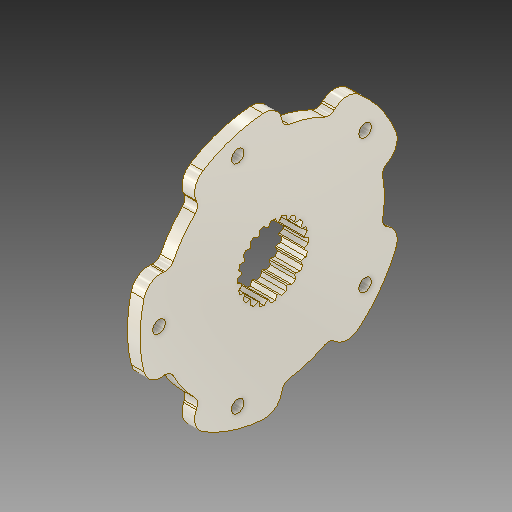
# Autodesk Inventor part: 362-04
Saved by Autodesk Inventor 2019 (Build 230136000, 136)
## iProperties
Company: Autodesk Inc.
Created: 2017-03-19
Part Number: 362-04
Material: Titanium
Document SubType Name: Modeling
Designer: Autodesk Inc.
Density: 4.51 g/cm^3
Appearance: Titanium - Polished
Mass: 217.983 g
Surface Area: 181.774 cm^2
Volume: 48.3334 cm^3
Author: Inventor
Autodesk Inventor part; units mm, degrees
ref_plane "YZ Plane" through (0, 0, 0) normal (1, 0, 0) x (0, 1, 0)
ref_plane "XZ Plane" through (0, 0, 0) normal (0, 1, 0) x (-1, 0, 0)
ref_plane "XY Plane" through (0, 0, 0) normal (0, 0, 1) x (1, 0, 0)
sketch "Sketch1" plane through (0, 0, 0) normal (1, 0, 0) x (0, 1, 0)
  arc A0 (12.5, 50.9902) -> (-12.5, 50.9902) centre (0, 0) ccw
  arc A1 (-19.5, 39.443) -> (-17.7114, 42.7254) centre (-20.9403, 42.3564) ccw
  line L0 (-17.7114, 42.7254) -> (-17.7881, 43.3968)
  arc A2 (-12.5, 50.9902) -> (-17.7881, 43.3968) centre (-10.8333, 44.1915) ccw
  line L1 (0, 0) -> (0, 52.5) construction
  arc A3 (17.7881, 43.3968) -> (12.5, 50.9902) centre (10.8333, 44.1915) ccw
  line L2 (17.7114, 42.7254) -> (17.7881, 43.3968)
  arc A4 (17.7114, 42.7254) -> (19.5, 39.443) centre (20.9403, 42.3564) ccw
  arc A5 (-44.6318, 27.645) -> (-52.3573, 3.8686) centre (0, 0) ccw
  arc A6 (-43.5384, -6.357) -> (-46.1074, -3.6416) centre (-46.7543, -6.8266) ccw
  line L3 (-46.1074, -3.6416) -> (-46.7696, -3.5071)
  arc A7 (-52.3573, 3.8686) -> (-46.7696, -3.5071) centre (-45.3763, 3.3528) ccw
  line L4 (0, 0) -> (-49.9305, 16.2234) construction
  arc A8 (-35.776, 30.3278) -> (-44.6318, 27.645) centre (-38.6809, 23.959) ccw
  line L5 (-35.1611, 30.0474) -> (-35.776, 30.3278)
  arc A9 (-35.1611, 30.0474) -> (-31.4867, 30.7342) centre (-33.8124, 33.0043) ccw
  arc A10 (-40.084, -33.9046) -> (-19.8586, -48.5993) centre (0, 0) ccw
  arc A11 (-7.4082, -43.3719) -> (-10.7846, -44.976) centre (-7.9554, -46.5755) ccw
  line L6 (-10.7846, -44.976) -> (-11.1171, -45.5643)
  arc A12 (-19.8586, -48.5993) -> (-11.1171, -45.5643) centre (-17.2108, -42.1194) ccw
  line L7 (0, 0) -> (-30.8587, -42.4734) construction
  arc A13 (-39.8989, -24.6532) -> (-40.084, -33.9046) centre (-34.7395, -29.384) ccw
  line L8 (-39.4421, -24.1551) -> (-39.8989, -24.6532)
  arc A14 (-39.4421, -24.1551) -> (-38.9598, -20.4482) centre (-41.8376, -21.9586) ccw
  arc A15 (19.8586, -48.5993) -> (40.084, -33.9046) centre (0, 0) ccw
  arc A16 (38.9598, -20.4482) -> (39.4421, -24.1551) centre (41.8376, -21.9586) ccw
  line L9 (39.4421, -24.1551) -> (39.8989, -24.6532)
  arc A17 (40.084, -33.9046) -> (39.8989, -24.6532) centre (34.7395, -29.384) ccw
  line L10 (0, 0) -> (30.8587, -42.4734) construction
  arc A18 (11.1171, -45.5643) -> (19.8586, -48.5993) centre (17.2108, -42.1194) ccw
  line L11 (10.7846, -44.976) -> (11.1171, -45.5643)
  arc A19 (10.7846, -44.976) -> (7.4082, -43.3719) centre (7.9554, -46.5755) ccw
  arc A20 (52.3573, 3.8686) -> (44.6318, 27.645) centre (0, 0) ccw
  arc A21 (31.4867, 30.7342) -> (35.1611, 30.0474) centre (33.8124, 33.0043) ccw
  line L12 (35.1611, 30.0474) -> (35.776, 30.3278)
  arc A22 (44.6318, 27.645) -> (35.776, 30.3278) centre (38.6809, 23.959) ccw
  line L13 (0, 0) -> (49.9305, 16.2234) construction
  arc A23 (46.7696, -3.5071) -> (52.3573, 3.8686) centre (45.3763, 3.3528) ccw
  line L14 (46.1074, -3.6416) -> (46.7696, -3.5071)
  arc A24 (46.1074, -3.6416) -> (43.5384, -6.357) centre (46.7543, -6.8266) ccw
  arc A25 (38.9598, -20.4482) -> (43.5384, -6.357) centre (0, 0) ccw
  arc A26 (-7.4082, -43.3719) -> (7.4082, -43.3719) centre (0, 0) ccw
  arc A27 (-43.5384, -6.357) -> (-38.9598, -20.4482) centre (0, 0) ccw
  arc A28 (31.4867, 30.7342) -> (19.5, 39.443) centre (0, 0) ccw
  arc A29 (-19.5, 39.443) -> (-31.4867, 30.7342) centre (0, 0) ccw
  dimension "d118" = 52.5
  dimension "d119" = 7
  dimension "d120" = 3.25
  dimension "d121" = 360
  dimension "d122" = 44
  dimension "d123" = 12.5
  dimension "d124" = 19.5
  constraints: 77 point on circle, 30 centre point, 30 end point, 6 symmetric about line, 5 coincident, 5 tangent, 1 vertical, 142 other
  measures "d118" radius of A0
  measures "d119" radius of A2
  measures "d120" radius of A1
  measures "d122" radius of A28
  measures "d123" distance from line of L1 A0.end
  measures "d124" distance from line of L1 A1.start
extrude "Extrusion1" add sketch "Sketch1" along normal blind 5
sketch "Sketch2" plane through (0, 0, 0) normal (-1, 0, 0) x (0, 0, 1)
  circle A0 centre (0, 0) radius 32.5
  dimension "d104" = 65
  constraints: 1 centre point, 1 coincident
  measures "d104" diameter of A0
extrude "Extrusion2" add sketch "Sketch2" along normal blind 5
sketch "Sketch3" plane through (5, 0, 0) normal (1, 0, 0) x (0, 0, -1)
  line L0 (0, -73.3268) -> (0, 73.3268) construction
  line L1 (69.4432, 0) -> (-72.8239, 0) construction
  circle A0 centre (-45, 0) radius 2.5
  point P0 (0, 0)
  dimension "d107" = 5
  dimension "d108" = 45
  constraints: 1 centre point, 1 point on line
  measures "d107" diameter of A0
  measures "d108" distance from line of L0 A0.centre
extrude "Extrusion3" cut sketch "Sketch3" against normal through all
pattern_circular "Circular Pattern1" count 5 over 360 about axis through (-10, 0, 0) along (1, 0, 0) of "Extrusion3"
sketch "Sketch4" plane through (5, 0, 0) normal (1, 0, 0) x (0, 0, -1)
  arc A0 (-5.4322, 11.258) -> (-5.9149, 11.012) centre (0, 0) ccw
  line L0 (0, -21) -> (0, 21) construction
  line L1 (-0.9, 14) -> (0.9, 14)
  line L2 (-0.9, 14) -> (-1.6874, 12.3856)
  line L3 (0.9, 14) -> (1.6874, 12.3856)
  line L4 (-5.1822, 13.0367) -> (-5.4322, 11.258)
  line L5 (-5.1822, 13.0367) -> (-3.4703, 13.5929)
  line L6 (-3.4703, 13.5929) -> (-2.2225, 12.3008)
  line L7 (-8.9571, 10.7972) -> (-8.6452, 9.0283)
  line L8 (-8.9571, 10.7972) -> (-7.5009, 11.8552)
  line L9 (-7.5009, 11.8552) -> (-5.9149, 11.012)
  line L10 (-11.8552, 7.5009) -> (-11.012, 5.9149)
  line L11 (-11.8552, 7.5009) -> (-10.7972, 8.9571)
  line L12 (-10.7972, 8.9571) -> (-9.0283, 8.6452)
  line L13 (-13.5929, 3.4703) -> (-12.3008, 2.2225)
  line L14 (-13.5929, 3.4703) -> (-13.0367, 5.1822)
  line L15 (-13.0367, 5.1822) -> (-11.258, 5.4322)
  line L16 (-14, -0.9) -> (-12.3856, -1.6874)
  line L17 (-14, -0.9) -> (-14, 0.9)
  line L18 (-14, 0.9) -> (-12.3856, 1.6874)
  line L19 (-13.0367, -5.1822) -> (-11.258, -5.4322)
  line L20 (-13.0367, -5.1822) -> (-13.5929, -3.4703)
  line L21 (-13.5929, -3.4703) -> (-12.3008, -2.2225)
  line L22 (-10.7972, -8.9571) -> (-9.0283, -8.6452)
  line L23 (-10.7972, -8.9571) -> (-11.8552, -7.5009)
  line L24 (-11.8552, -7.5009) -> (-11.012, -5.9149)
  line L25 (-7.5009, -11.8552) -> (-5.9149, -11.012)
  line L26 (-7.5009, -11.8552) -> (-8.9571, -10.7972)
  line L27 (-8.9571, -10.7972) -> (-8.6452, -9.0283)
  line L28 (-3.4703, -13.5929) -> (-2.2225, -12.3008)
  line L29 (-3.4703, -13.5929) -> (-5.1822, -13.0367)
  line L30 (-5.1822, -13.0367) -> (-5.4322, -11.258)
  line L31 (0.9, -14) -> (1.6874, -12.3856)
  line L32 (0.9, -14) -> (-0.9, -14)
  line L33 (-0.9, -14) -> (-1.6874, -12.3856)
  line L34 (5.1822, -13.0367) -> (5.4322, -11.258)
  line L35 (5.1822, -13.0367) -> (3.4703, -13.5929)
  line L36 (3.4703, -13.5929) -> (2.2225, -12.3008)
  line L37 (8.9571, -10.7972) -> (8.6452, -9.0283)
  line L38 (8.9571, -10.7972) -> (7.5009, -11.8552)
  line L39 (7.5009, -11.8552) -> (5.9149, -11.012)
  line L40 (11.8552, -7.5009) -> (11.012, -5.9149)
  line L41 (11.8552, -7.5009) -> (10.7972, -8.9571)
  line L42 (10.7972, -8.9571) -> (9.0283, -8.6452)
  line L43 (13.5929, -3.4703) -> (12.3008, -2.2225)
  line L44 (13.5929, -3.4703) -> (13.0367, -5.1822)
  line L45 (13.0367, -5.1822) -> (11.258, -5.4322)
  line L46 (14, 0.9) -> (12.3856, 1.6874)
  line L47 (14, 0.9) -> (14, -0.9)
  line L48 (14, -0.9) -> (12.3856, -1.6874)
  line L49 (13.0367, 5.1822) -> (11.258, 5.4322)
  line L50 (13.0367, 5.1822) -> (13.5929, 3.4703)
  line L51 (13.5929, 3.4703) -> (12.3008, 2.2225)
  line L52 (10.7972, 8.9571) -> (9.0283, 8.6452)
  line L53 (10.7972, 8.9571) -> (11.8552, 7.5009)
  line L54 (11.8552, 7.5009) -> (11.012, 5.9149)
  line L55 (7.5009, 11.8552) -> (5.9149, 11.012)
  line L56 (7.5009, 11.8552) -> (8.9571, 10.7972)
  line L57 (8.9571, 10.7972) -> (8.6452, 9.0283)
  line L58 (3.4703, 13.5929) -> (2.2225, 12.3008)
  line L59 (3.4703, 13.5929) -> (5.1822, 13.0367)
  line L60 (5.1822, 13.0367) -> (5.4322, 11.258)
  arc A1 (-2.2225, 12.3008) -> (-5.4322, 11.258) centre (0, 0) ccw
  arc A2 (-5.9149, 11.012) -> (-8.6452, 9.0283) centre (0, 0) ccw
  arc A3 (-8.6452, 9.0283) -> (-9.0283, 8.6452) centre (0, 0) ccw
  arc A4 (-9.0283, 8.6452) -> (-11.012, 5.9149) centre (0, 0) ccw
  arc A5 (-11.012, 5.9149) -> (-11.258, 5.4322) centre (0, 0) ccw
  arc A6 (-11.258, 5.4322) -> (-12.3008, 2.2225) centre (0, 0) ccw
  arc A7 (-12.3008, 2.2225) -> (-12.3856, 1.6874) centre (0, 0) ccw
  arc A8 (-12.3856, 1.6874) -> (-12.3856, -1.6874) centre (0, 0) ccw
  arc A9 (-12.3856, -1.6874) -> (-12.3008, -2.2225) centre (0, 0) ccw
  arc A10 (-12.3008, -2.2225) -> (-11.258, -5.4322) centre (0, 0) ccw
  arc A11 (-11.258, -5.4322) -> (-11.012, -5.9149) centre (0, 0) ccw
  arc A12 (-11.012, -5.9149) -> (-9.0283, -8.6452) centre (0, 0) ccw
  arc A13 (-8.6452, -9.0283) -> (-5.9149, -11.012) centre (0, 0) ccw
  arc A14 (-5.9149, -11.012) -> (-5.4322, -11.258) centre (0, 0) ccw
  arc A15 (-5.4322, -11.258) -> (-2.2225, -12.3008) centre (0, 0) ccw
  arc A16 (-2.2225, -12.3008) -> (-1.6874, -12.3856) centre (0, 0) ccw
  arc A17 (-1.6874, -12.3856) -> (1.6874, -12.3856) centre (0, 0) ccw
  arc A18 (1.6874, -12.3856) -> (2.2225, -12.3008) centre (0, 0) ccw
  arc A19 (2.2225, -12.3008) -> (5.4322, -11.258) centre (0, 0) ccw
  arc A20 (5.4322, -11.258) -> (5.9149, -11.012) centre (0, 0) ccw
  arc A21 (5.9149, -11.012) -> (8.6452, -9.0283) centre (0, 0) ccw
  arc A22 (8.6452, -9.0283) -> (9.0283, -8.6452) centre (0, 0) ccw
  arc A23 (9.0283, -8.6452) -> (11.012, -5.9149) centre (0, 0) ccw
  arc A24 (11.012, -5.9149) -> (11.258, -5.4322) centre (0, 0) ccw
  arc A25 (11.258, -5.4322) -> (12.3008, -2.2225) centre (0, 0) ccw
  arc A26 (12.3008, -2.2225) -> (12.3856, -1.6874) centre (0, 0) ccw
  arc A27 (12.3856, -1.6874) -> (12.3856, 1.6874) centre (0, 0) ccw
  arc A28 (12.3856, 1.6874) -> (12.3008, 2.2225) centre (0, 0) ccw
  arc A29 (11.258, 5.4322) -> (11.012, 5.9149) centre (0, 0) ccw
  arc A30 (12.3008, 2.2225) -> (11.258, 5.4322) centre (0, 0) ccw
  arc A31 (11.012, 5.9149) -> (9.0283, 8.6452) centre (0, 0) ccw
  arc A32 (9.0283, 8.6452) -> (8.6452, 9.0283) centre (0, 0) ccw
  arc A33 (5.9149, 11.012) -> (5.4322, 11.258) centre (0, 0) ccw
  arc A34 (8.6452, 9.0283) -> (5.9149, 11.012) centre (0, 0) ccw
  arc A35 (2.2225, 12.3008) -> (1.6874, 12.3856) centre (0, 0) ccw
  arc A36 (5.4322, 11.258) -> (2.2225, 12.3008) centre (0, 0) ccw
  arc A37 (1.6874, 12.3856) -> (-1.6874, 12.3856) centre (0, 0) ccw
  arc A38 (-1.6874, 12.3856) -> (-2.2225, 12.3008) centre (0, 0) ccw
  arc A39 (-9.0283, -8.6452) -> (-8.6452, -9.0283) centre (0, 0) ccw
  point P0 (0, 14)
  point P1 (-4.3262, 13.3148)
  point P2 (-8.229, 11.3262)
  point P3 (-11.3262, 8.229)
  point P4 (-13.3148, 4.3262)
  point P5 (-14, 0)
  point P6 (-13.3148, -4.3262)
  point P7 (-11.3262, -8.229)
  point P8 (-8.229, -11.3262)
  point P9 (-4.3262, -13.3148)
  point P10 (0, -14)
  point P11 (4.3262, -13.3148)
  point P12 (8.229, -11.3262)
  point P13 (11.3262, -8.229)
  point P14 (13.3148, -4.3262)
  point P15 (14, 0)
  point P16 (13.3148, 4.3262)
  point P17 (11.3262, 8.229)
  point P18 (8.229, 11.3262)
  point P19 (4.3262, 13.3148)
  dimension "d127" = 25
  dimension "d128" = 1.8
  dimension "d129" = 14
  dimension "d130" = 116
  dimension "d131" = 360
  constraints: 120 end point, 2 vertical alignment, 1 horizontal, 1 horizontal alignment, 1 midpoint, 1 point on line, 278 other
  measures "d128" distance of L1.start L1.end
  measures "d129" distance from line of point (0, 0) L1
  measures "d130" angle of L1 L2
extrude "Extrusion4" cut sketch "Sketch4" against normal through all
body "Solid1"
